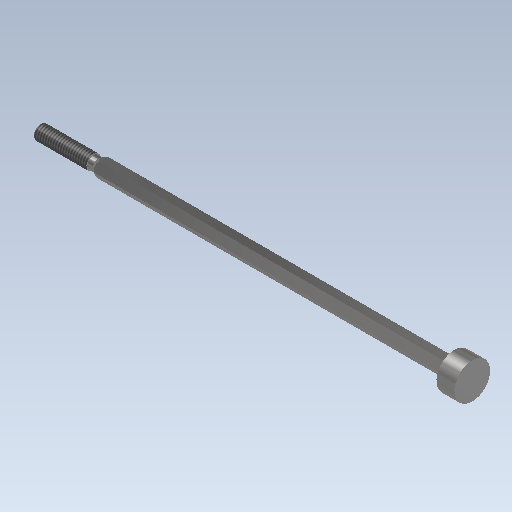
# Autodesk Inventor part: CJ2KB10-75Z_ROD
Saved by Autodesk Inventor 2021.3 (Build 253353010, 353A)
## iProperties
Created: 2019-10-24
Part Number: CJ2KB10-75Z_ROD
Material: ステンレス鋼
Catalog Web Link: www.cadenas.de
Description: CJ2K-Z_ROD-Air Cylinder/Non-rotating Rod Type: Double Acting, Single Rod
Vendor: SMC
Document SubType Name: Modeling
Designer: psadmin
Manufacturer: SMC
Mass: 16.8361 g
Surface Area: 19.5604 cm^2
Volume: 2.10452 cm^3
Density: 8 g/cm^3
Appearance: 半つや出し
Category: PARTsolutions
Company: SMC
PSOL_IDENT_0: {$CADENAS_DATA\23d-libs\smc_jp\actuator\standard_air_cylinder\cj2\cj2k_z\parts\cj2k_z_rod.prj},187 {
PSOL_IDENT_1: VTYP=3D},{NB=CJ2KB10-75Z_ROD},{LINA=CJ2KB10-75Z_ROD},{NN=CJ2K-Z_ROD},{DATE=07.02.2019 07:32:01},{GEO
PSOL_IDENT_2: MDATE=08.04.2018 05:08:15},{VERSION=},{LINEID=370},{WBVAR=STROKE},{WBNUMERIC=STROKE}  {NB=CJ2KB10-75
PSOL_IDENT_3: Z_ROD},{LINA=CJ2KB10-75Z_ROD},{KT=DUMMY},{ORDER=CJ2KB10-75Z},{BORE=10},{MOUNT=(B) Basic},{MOUNTX=B},
PSOL_IDENT_4: {STROKE=75},{A=15},{F=8.0},{H=28},{KA=4.2},{MM=M4x0.7},{MM1=4},{MM2=0.7},{NA=12.5}
NN: CJ2K-Z_ROD
NT: Air Cylinder/Non-rotating Rod Type: Double Acting, Single Rod
NB: CJ2KB10-75Z_ROD
NBSYN: $ORDER._ROD
LINA: CJ2KB10-75Z_ROD
BORE: 10
MOUNT: (B) Basic
MOUNTX: B
STROKE: 75
A: 15
F: 8
H: 28
KA: 4.2
MM: M4x0.7
MM1: 4
MM2: 0.7
NA: 12.5
SUPPLIER: SMC
ARTICLENO: CJ2KB10-75Z_ROD
BOMINFO: CJ2KB10-75Z_ROD
CREATOR: CADENAS GmbH
Title: CJ2KB10-75Z_ROD
Author: Cadenas PARTsolutions
Comments: Air Cylinder/Non-rotating Rod Type: Double Acting, Single Rod
Autodesk Inventor part; units mm, degrees
sketch "Sketch_2" plane through (0, 0, 0) normal (0, 0, 1) x (1, 0, 0)
  line L0 (120.5, 0) -> (0, 0)
  line L1 (0, 0) -> (0, 1.5705)
  line L2 (0, 1.5705) -> (0.4295, 2)
  line L3 (0.4295, 2) -> (15, 2)
  line L4 (15, 2) -> (15, 1.75)
  line L5 (15, 1.75) -> (16.5, 1.75)
  line L6 (16.5, 1.75) -> (17.6689, 2.4249)
  line L7 (17.6689, 2.4249) -> (115.5, 2.4249)
  line L8 (115.5, 2.4249) -> (115.5, 5)
  line L9 (115.5, 5) -> (120.5, 5)
  line L10 (120.5, 5) -> (120.5, 0)
  line L11 (120.5, 0) -> (0, 0)
  constraints: 24 end point
revolve "Revolution1" add sketch "Sketch_2" angle 360 about axis through (120.5, 0, 0) along (1, 0, 0)
thread "Thread1" size "M4x0.7" class "6g" standard "ISO Metric profile" full length
sketch "Sketch_1" plane through (15, 0, 0) normal (1, 0, 0) x (0, 0, -1)
  circle A0 centre (0, 0) radius 6.3
  line L0 (-2.4249, 0) -> (-1.2124, -2.1)
  line L1 (-1.2124, -2.1) -> (1.2124, -2.1)
  line L2 (1.2124, -2.1) -> (2.4249, 0)
  line L3 (2.4249, 0) -> (1.2124, 2.1)
  line L4 (1.2124, 2.1) -> (-1.2124, 2.1)
  line L5 (-1.2124, 2.1) -> (-2.4249, 0)
  constraints: 12 end point, 1 centre point
extrude "Extrusion1" cut sketch "Sketch_1" along normal blind 100.5
ref_plane "rod_XY" through (0, 0, 0) normal (1, 0, 0) x (0, 0, -1)
ref_plane "rod_YZ" through (0, 0, 0) normal (0, 0, -1) x (0, 1, 0)
ref_plane "rod_ZX" through (0, 0, 0) normal (0, 1, 0) x (1, 0, 0)
ref_plane "rodnt1_XY" through (7.5, 0, 0) normal (1, 0, 0) x (0, 0, -1)
ref_plane "rodnt1_YZ" through (7.5, 0, 0) normal (0, 0, -1) x (0, 1, 0)
ref_plane "rodnt1_ZX" through (7.5, 0, 0) normal (0, 1, 0) x (1, 0, 0)
ref_plane "rodnt2_XY" through (7.5, 0, 0) normal (-1, 0, 0) x (0, 0, -1)
ref_plane "rodnt2_YZ" through (7.5, 0, 0) normal (0, 0, -1) x (0, -1, 0)
ref_plane "rodnt2_ZX" through (7.5, 0, 0) normal (0, -1, 0) x (-1, 0, 0)
body "Solid1"
